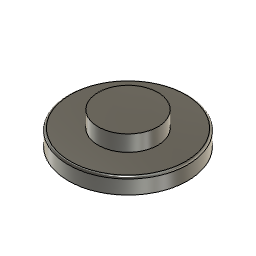
ROBOTIC ARM v2 (Autodesk Fusion 360 design; units mm, degrees)
Autodesk Fusion 360 part; units mm, degrees
sketch "Sketch1" plane through (0, 0, 0) normal (0, 0, 1) x (1, 0, 0)
  circle A0 centre (0, 0) radius 150
  constraint coincident A0.centre origin
extrude "Extrude1" add sketch "Sketch1" along normal blind 40
sketch "Sketch2" plane through (0, 0, 40) normal (0, 0, 1) x (-1, 0, 0)
  circle A0 centre (0, 0) radius 150
  circle A1 centre (0, 0) radius 75
  constraint coincident A0.centre A1.centre
extrude "Extrude2" add sketch "Sketch2" along normal blind 40 contours A1
fillet "Fillet1" radius 5 1 edges at (-139.8491, -54.2423, 40)
